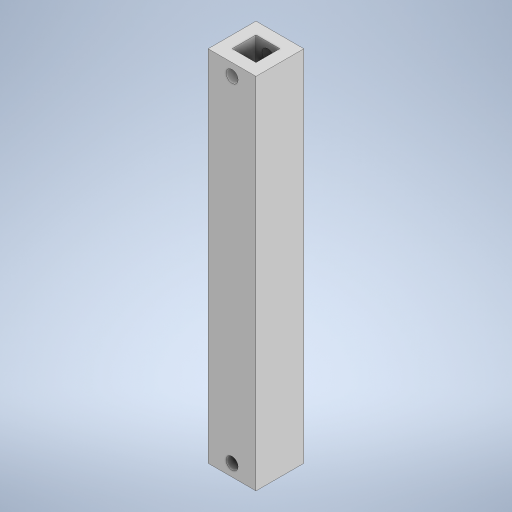
# Autodesk Inventor part: asta
Saved by Autodesk Inventor 2023 (Build 270158000, 158)
## iProperties
Created: 2023-08-01
Part Number: asta
Material: Generico
Document SubType Name: Modeling
Designer: Admin
Density: 1 g/cm^3
Appearance: Default
Author: Admin
Autodesk Inventor part; units mm, degrees
ref_plane "YZ Plane" through (0, 0, 0) normal (1, 0, 0) x (0, 1, 0)
ref_plane "XZ Plane" through (0, 0, 0) normal (0, 1, 0) x (-1, 0, 0)
ref_plane "XY Plane" through (0, 0, 0) normal (0, 0, 1) x (1, 0, 0)
sketch "Schizzo2" plane through (0, 0, 0) normal (0, 1, 0) x (-1, 0, 0)
  line L0 (10, 10) -> (-10, 10)
  line L1 (-10, 10) -> (-10, -10)
  line L2 (-10, -10) -> (10, -10)
  line L3 (10, -10) -> (10, 10)
  line L4 (0, 0) -> (12.3098, 0) construction
  line L5 (0, 0) -> (0, -18.6141) construction
  line L6 (5, 5) -> (-5, 5)
  line L7 (-5, 5) -> (-5, -5)
  line L8 (-5, -5) -> (5, -5)
  line L9 (5, -5) -> (5, 5)
  dimension "d0" = 20
  dimension "d1" = 5
  constraints: 20 end point, 4 parallel, 3 perpendicular, 2 horizontal, 1 vertical, 5 other
  measures "d0" distance of L2.end L0.start
  measures "d1" distance between parallel lines of L3 L9
extrude "Estrusione1" add sketch "Schizzo2" along normal mid plane 150
sketch "Schizzo3" plane through (0, 0, 0) normal (0, 0, 1) x (1, 0, 0)
  line L0 (-10, -75) -> (-10, 75) projected
  line L1 (10, -75) -> (-10, -75) projected
  line L2 (-10, 75) -> (10, 75) projected
  line L3 (10, 75) -> (10, -75) projected
  line L4 (0, 0) -> (0, 99.3871) construction
  line L5 (0, 0) -> (72.2632, 0) construction
  circle A0 centre (0, 70) radius 2.5
  circle A1 centre (0, -70) radius 2.5
  circle A2 centre (0, 60) radius 2.5
  dimension "d4" = 5
  dimension "d5" = 5
  dimension "d8" = 5
  dimension "d9" = 10
  constraints: 4 end point, 3 centre point, 2 point on line, 1 horizontal, 1 symmetric about line, 1 vertical, 1 other
  measures "d4" diameter of A0
  measures "d5" distance from line of A0.centre L2
  measures "d8" diameter of A2
  measures "d9" distance of A2.centre A0.centre
extrude "Estrusione2" cut sketch "Schizzo3" along normal through all both and the other way through all contours A0 | A1
